Autodesk Fusion 360 part; units mm, degrees
(part 3 of 6)
sketch "b bottom  projection" plane through (0, 0, 0) normal (0, 0, 1) x (1, 0, 0) in component "b bottom component"
  arc A0 (298.8505, 15.08) -> (300.4408, 15.08) centre (299.6456, 15.6946) ccw
  arc A1 (300.4408, 24.92) -> (298.8505, 24.92) centre (299.6456, 24.3054) ccw
  arc A2 (298.835, 24.8994) -> (298.835, 23.7113) centre (299.6456, 24.3054) ccw
  arc A3 (291.9094, 3.175) -> (290.7213, 3.175) centre (291.3154, 2.3644) ccw
  arc A4 (291.93, 1.5692) -> (291.93, 3.1595) centre (291.3154, 2.3644) ccw
  arc A5 (298.835, 36.2887) -> (298.835, 35.1006) centre (299.6456, 35.6946) ccw
  arc A6 (298.8505, 35.08) -> (300.4408, 35.08) centre (299.6456, 35.6946) ccw
  arc A7 (282.09, 3.1595) -> (282.09, 1.5692) centre (282.7046, 2.3644) ccw
  arc A8 (283.2987, 3.175) -> (282.1106, 3.175) centre (282.7046, 2.3644) ccw
  arc A9 (300.4408, 44.92) -> (298.8505, 44.92) centre (299.6456, 44.3054) ccw
  arc A10 (298.835, 44.8994) -> (298.835, 43.7113) centre (299.6456, 44.3054) ccw
  arc A11 (271.9094, 3.175) -> (270.7213, 3.175) centre (271.3154, 2.3644) ccw
  arc A12 (271.93, 1.5692) -> (271.93, 3.1595) centre (271.3154, 2.3644) ccw
  arc A13 (298.835, 56.2887) -> (298.835, 55.1006) centre (299.6456, 55.6946) ccw
  arc A14 (298.8505, 55.08) -> (300.4408, 55.08) centre (299.6456, 55.6946) ccw
  arc A15 (262.09, 3.1595) -> (262.09, 1.5692) centre (262.7046, 2.3644) ccw
  arc A16 (263.2987, 3.175) -> (262.1106, 3.175) centre (262.7046, 2.3644) ccw
  arc A17 (300.4408, 64.92) -> (298.8505, 64.92) centre (299.6456, 64.3054) ccw
  arc A18 (298.835, 64.8994) -> (298.835, 63.7113) centre (299.6456, 64.3054) ccw
  arc A19 (251.9094, 3.175) -> (250.7213, 3.175) centre (251.3154, 2.3644) ccw
  arc A20 (251.93, 1.5692) -> (251.93, 3.1595) centre (251.3154, 2.3644) ccw
  arc A21 (298.835, 76.2887) -> (298.835, 75.1006) centre (299.6456, 75.6946) ccw
  arc A22 (298.8505, 75.08) -> (300.4408, 75.08) centre (299.6456, 75.6946) ccw
  arc A23 (242.09, 3.1595) -> (242.09, 1.5692) centre (242.7046, 2.3644) ccw
  arc A24 (243.2987, 3.175) -> (242.1106, 3.175) centre (242.7046, 2.3644) ccw
  arc A25 (300.4408, 84.92) -> (298.8505, 84.92) centre (299.6456, 84.3054) ccw
  arc A26 (298.835, 84.8994) -> (298.835, 83.7113) centre (299.6456, 84.3054) ccw
  arc A27 (231.9094, 3.175) -> (230.7213, 3.175) centre (231.3154, 2.3644) ccw
  arc A28 (231.93, 1.5692) -> (231.93, 3.1595) centre (231.3154, 2.3644) ccw
  arc A29 (222.09, 3.1595) -> (222.09, 1.5692) centre (222.7046, 2.3644) ccw
  arc A30 (223.2987, 3.175) -> (222.1106, 3.175) centre (222.7046, 2.3644) ccw
  arc A31 (298.835, 96.2887) -> (298.835, 95.1006) centre (299.6456, 95.6946) ccw
  arc A32 (298.8505, 95.08) -> (300.4408, 95.08) centre (299.6456, 95.6946) ccw
  arc A33 (300.4408, 104.92) -> (298.8505, 104.92) centre (299.6456, 104.3054) ccw
  arc A34 (298.835, 104.8994) -> (298.835, 103.7113) centre (299.6456, 104.3054) ccw
  arc A35 (211.9094, 3.175) -> (210.7213, 3.175) centre (211.3154, 2.3644) ccw
  arc A36 (211.93, 1.5692) -> (211.93, 3.1595) centre (211.3154, 2.3644) ccw
  arc A37 (202.09, 3.1595) -> (202.09, 1.5692) centre (202.7046, 2.3644) ccw
  arc A38 (203.2987, 3.175) -> (202.1106, 3.175) centre (202.7046, 2.3644) ccw
  arc A39 (290.7213, 116.825) -> (291.9094, 116.825) centre (291.3154, 117.6356) ccw
  arc A40 (291.93, 116.8405) -> (291.93, 118.4308) centre (291.3154, 117.6356) ccw
  arc A41 (191.9094, 3.175) -> (190.7213, 3.175) centre (191.3154, 2.3644) ccw
  arc A42 (191.93, 1.5692) -> (191.93, 3.1595) centre (191.3154, 2.3644) ccw
  arc A43 (282.09, 118.4308) -> (282.09, 116.8405) centre (282.7046, 117.6356) ccw
  arc A44 (282.1106, 116.825) -> (283.2987, 116.825) centre (282.7046, 117.6356) ccw
  arc A45 (182.09, 3.1595) -> (182.09, 1.5692) centre (182.7046, 2.3644) ccw
  arc A46 (183.2987, 3.175) -> (182.1106, 3.175) centre (182.7046, 2.3644) ccw
  arc A47 (270.7213, 116.825) -> (271.9094, 116.825) centre (271.3154, 117.6356) ccw
  arc A48 (271.93, 116.8405) -> (271.93, 118.4308) centre (271.3154, 117.6356) ccw
  arc A49 (171.9094, 3.175) -> (170.7213, 3.175) centre (171.3154, 2.3644) ccw
  arc A50 (171.93, 1.5692) -> (171.93, 3.1595) centre (171.3154, 2.3644) ccw
  arc A51 (262.09, 118.4308) -> (262.09, 116.8405) centre (262.7046, 117.6356) ccw
  arc A52 (262.1106, 116.825) -> (263.2987, 116.825) centre (262.7046, 117.6356) ccw
  arc A53 (162.09, 3.1595) -> (162.09, 1.5692) centre (162.7046, 2.3644) ccw
  arc A54 (163.2987, 3.175) -> (162.1106, 3.175) centre (162.7046, 2.3644) ccw
  arc A55 (250.7213, 116.825) -> (251.9094, 116.825) centre (251.3154, 117.6356) ccw
  arc A56 (251.93, 116.8405) -> (251.93, 118.4308) centre (251.3154, 117.6356) ccw
  arc A57 (242.09, 118.4308) -> (242.09, 116.8405) centre (242.7046, 117.6356) ccw
  arc A58 (242.1106, 116.825) -> (243.2987, 116.825) centre (242.7046, 117.6356) ccw
  arc A59 (155.185, 15.1006) -> (155.185, 16.2887) centre (154.3744, 15.6946) ccw
  arc A60 (153.5792, 15.08) -> (155.1695, 15.08) centre (154.3744, 15.6946) ccw
  arc A61 (155.1695, 24.92) -> (153.5792, 24.92) centre (154.3744, 24.3054) ccw
  arc A62 (155.185, 23.7113) -> (155.185, 24.8994) centre (154.3744, 24.3054) ccw
  arc A63 (230.7213, 116.825) -> (231.9094, 116.825) centre (231.3154, 117.6356) ccw
  arc A64 (231.93, 116.8405) -> (231.93, 118.4308) centre (231.3154, 117.6356) ccw
  arc A65 (155.185, 35.1006) -> (155.185, 36.2887) centre (154.3744, 35.6946) ccw
  arc A66 (153.5792, 35.08) -> (155.1695, 35.08) centre (154.3744, 35.6946) ccw
  arc A67 (222.09, 118.4308) -> (222.09, 116.8405) centre (222.7046, 117.6356) ccw
  arc A68 (222.1106, 116.825) -> (223.2987, 116.825) centre (222.7046, 117.6356) ccw
  arc A69 (155.1695, 44.92) -> (153.5792, 44.92) centre (154.3744, 44.3054) ccw
  arc A70 (155.185, 43.7113) -> (155.185, 44.8994) centre (154.3744, 44.3054) ccw
  arc A71 (210.7213, 116.825) -> (211.9094, 116.825) centre (211.3154, 117.6356) ccw
  arc A72 (211.93, 116.8405) -> (211.93, 118.4308) centre (211.3154, 117.6356) ccw
  arc A73 (155.185, 55.1006) -> (155.185, 56.2887) centre (154.3744, 55.6946) ccw
  arc A74 (153.5792, 55.08) -> (155.1695, 55.08) centre (154.3744, 55.6946) ccw
  arc A75 (202.09, 118.4308) -> (202.09, 116.8405) centre (202.7046, 117.6356) ccw
  arc A76 (202.1106, 116.825) -> (203.2987, 116.825) centre (202.7046, 117.6356) ccw
  arc A77 (155.1695, 64.92) -> (153.5792, 64.92) centre (154.3744, 64.3054) ccw
  arc A78 (155.185, 63.7113) -> (155.185, 64.8994) centre (154.3744, 64.3054) ccw
  arc A79 (190.7213, 116.825) -> (191.9094, 116.825) centre (191.3154, 117.6356) ccw
  arc A80 (191.93, 116.8405) -> (191.93, 118.4308) centre (191.3154, 117.6356) ccw
  arc A81 (155.185, 75.1006) -> (155.185, 76.2887) centre (154.3744, 75.6946) ccw
  arc A82 (153.5792, 75.08) -> (155.1695, 75.08) centre (154.3744, 75.6946) ccw
  arc A83 (182.09, 118.4308) -> (182.09, 116.8405) centre (182.7046, 117.6356) ccw
  arc A84 (182.1106, 116.825) -> (183.2987, 116.825) centre (182.7046, 117.6356) ccw
  arc A85 (155.1695, 84.92) -> (153.5792, 84.92) centre (154.3744, 84.3054) ccw
  arc A86 (155.185, 83.7113) -> (155.185, 84.8994) centre (154.3744, 84.3054) ccw
  arc A87 (170.7213, 116.825) -> (171.9094, 116.825) centre (171.3154, 117.6356) ccw
  arc A88 (171.93, 116.8405) -> (171.93, 118.4308) centre (171.3154, 117.6356) ccw
  arc A89 (155.185, 95.1006) -> (155.185, 96.2887) centre (154.3744, 95.6946) ccw
  arc A90 (153.5792, 95.08) -> (155.1695, 95.08) centre (154.3744, 95.6946) ccw
  arc A91 (162.09, 118.4308) -> (162.09, 116.8405) centre (162.7046, 117.6356) ccw
  arc A92 (162.1106, 116.825) -> (163.2987, 116.825) centre (162.7046, 117.6356) ccw
  arc A93 (155.1695, 104.92) -> (153.5792, 104.92) centre (154.3744, 104.3054) ccw
  arc A94 (155.185, 103.7113) -> (155.185, 104.8994) centre (154.3744, 104.3054) ccw
  arc A95 (298.835, 16.2887) -> (298.835, 15.1006) centre (299.6456, 15.6946) ccw
  line L0 (302.01, 15.08) -> (300.4408, 15.08)
  line L1 (298.835, 24.8994) -> (298.835, 24.92)
  line L2 (298.835, 16.2887) -> (298.835, 23.7113)
  line L3 (298.835, 15.08) -> (298.835, 15.1006)
  line L4 (300.4408, 24.92) -> (302.01, 24.92)
  line L5 (291.93, 3.175) -> (291.93, 3.1595)
  line L6 (298.8505, 35.08) -> (298.835, 35.08)
  line L7 (282.09, 3.175) -> (282.1106, 3.175)
  line L8 (283.2987, 3.175) -> (290.7213, 3.175)
  line L9 (282.09, 0) -> (282.09, 1.5692)
  line L10 (298.835, 44.8994) -> (298.835, 44.92)
  line L11 (298.835, 36.2887) -> (298.835, 43.7113)
  line L12 (300.4408, 44.92) -> (302.01, 44.92)
  line L13 (271.93, 3.175) -> (271.93, 3.1595)
  line L14 (298.8505, 55.08) -> (298.835, 55.08)
  line L15 (262.09, 3.175) -> (262.1106, 3.175)
  line L16 (263.2987, 3.175) -> (270.7213, 3.175)
  line L17 (262.09, 0) -> (262.09, 1.5692)
  line L18 (298.835, 64.8994) -> (298.835, 64.92)
  line L19 (298.835, 56.2887) -> (298.835, 63.7113)
  line L20 (251.93, 3.175) -> (251.93, 3.1595)
  line L21 (300.4408, 64.92) -> (302.01, 64.92)
  line L22 (298.8505, 75.08) -> (298.835, 75.08)
  line L23 (242.09, 3.175) -> (242.1106, 3.175)
  line L24 (243.2987, 3.175) -> (250.7213, 3.175)
  line L25 (242.09, 0) -> (242.09, 1.5692)
  line L26 (298.835, 84.8994) -> (298.835, 84.92)
  line L27 (298.835, 76.2887) -> (298.835, 83.7113)
  line L28 (231.93, 3.175) -> (231.93, 3.1595)
  line L29 (300.4408, 84.92) -> (302.01, 84.92)
  line L30 (222.09, 3.175) -> (222.1106, 3.175)
  line L31 (223.2987, 3.175) -> (230.7213, 3.175)
  line L32 (298.8505, 95.08) -> (298.835, 95.08)
  line L33 (222.09, 0) -> (222.09, 1.5692)
  line L34 (298.835, 104.8994) -> (298.835, 104.92)
  line L35 (298.835, 96.2887) -> (298.835, 103.7113)
  line L36 (211.93, 3.175) -> (211.93, 3.1595)
  line L37 (300.4408, 104.92) -> (302.01, 104.92)
  line L38 (202.09, 3.175) -> (202.1106, 3.175)
  line L39 (203.2987, 3.175) -> (210.7213, 3.175)
  line L40 (291.93, 116.825) -> (291.93, 116.8405)
  line L41 (202.09, 0) -> (202.09, 1.5692)
  line L42 (282.09, 116.825) -> (282.1106, 116.825)
  line L43 (283.2987, 116.825) -> (290.7213, 116.825)
  line L44 (191.93, 3.175) -> (191.93, 3.1595)
  line L45 (282.09, 120) -> (282.09, 118.4308)
  line L46 (182.09, 3.175) -> (182.1106, 3.175)
  line L47 (183.2987, 3.175) -> (190.7213, 3.175)
  line L48 (271.93, 116.825) -> (271.93, 116.8405)
  line L49 (182.09, 0) -> (182.09, 1.5692)
  line L50 (262.09, 116.825) -> (262.1106, 116.825)
  line L51 (263.2987, 116.825) -> (270.7213, 116.825)
  line L52 (171.93, 3.175) -> (171.93, 3.1595)
  line L53 (262.09, 120) -> (262.09, 118.4308)
  line L54 (162.09, 3.175) -> (162.1106, 3.175)
  line L55 (163.2987, 3.175) -> (170.7213, 3.175)
  line L56 (251.93, 116.825) -> (251.93, 116.8405)
  line L57 (162.09, 0) -> (162.09, 1.5692)
  line L58 (242.09, 116.825) -> (242.1106, 116.825)
  line L59 (243.2987, 116.825) -> (250.7213, 116.825)
  line L60 (155.1695, 15.08) -> (155.185, 15.08)
  line L61 (242.09, 120) -> (242.09, 118.4308)
  line L62 (155.185, 24.8994) -> (155.185, 24.92)
  line L63 (155.185, 16.2887) -> (155.185, 23.7113)
  line L64 (231.93, 116.825) -> (231.93, 116.8405)
  line L65 (153.5792, 24.92) -> (152.01, 24.92)
  line L66 (222.09, 116.825) -> (222.1106, 116.825)
  line L67 (223.2987, 116.825) -> (230.7213, 116.825)
  line L68 (155.1695, 35.08) -> (155.185, 35.08)
  line L69 (222.09, 120) -> (222.09, 118.4308)
  line L70 (155.185, 44.8994) -> (155.185, 44.92)
  line L71 (155.185, 36.2887) -> (155.185, 43.7113)
  line L72 (211.93, 116.825) -> (211.93, 116.8405)
  line L73 (153.5792, 44.92) -> (152.01, 44.92)
  line L74 (155.1695, 55.08) -> (155.185, 55.08)
  line L75 (202.09, 116.825) -> (202.1106, 116.825)
  line L76 (203.2987, 116.825) -> (210.7213, 116.825)
  line L77 (202.09, 120) -> (202.09, 118.4308)
  line L78 (155.185, 64.8994) -> (155.185, 64.92)
  line L79 (155.185, 56.2887) -> (155.185, 63.7113)
  line L80 (153.5792, 64.92) -> (152.01, 64.92)
  line L81 (191.93, 116.825) -> (191.93, 116.8405)
  line L82 (155.1695, 75.08) -> (155.185, 75.08)
  line L83 (182.09, 116.825) -> (182.1106, 116.825)
  line L84 (183.2987, 116.825) -> (190.7213, 116.825)
  line L85 (155.185, 84.8994) -> (155.185, 84.92)
  line L86 (155.185, 76.2887) -> (155.185, 83.7113)
  line L87 (182.09, 120) -> (182.09, 118.4308)
  line L88 (153.5792, 84.92) -> (152.01, 84.92)
  line L89 (171.93, 116.825) -> (171.93, 116.8405)
  line L90 (155.1695, 95.08) -> (155.185, 95.08)
  line L91 (162.09, 116.825) -> (162.1106, 116.825)
  line L92 (163.2987, 116.825) -> (170.7213, 116.825)
  line L93 (155.185, 104.8994) -> (155.185, 104.92)
  line L94 (155.185, 96.2887) -> (155.185, 103.7113)
  line L95 (162.09, 120) -> (162.09, 118.4308)
  line L96 (153.5792, 104.92) -> (152.01, 104.92)
  line L97 (152.01, 0) -> (152.01, 15.08)
  line L98 (152.01, 15.08) -> (153.5792, 15.08)
  line L99 (155.185, 15.08) -> (155.185, 15.1006)
  line L100 (155.185, 24.92) -> (155.1695, 24.92)
  line L101 (152.01, 24.92) -> (152.01, 35.08)
  line L102 (152.01, 35.08) -> (153.5792, 35.08)
  line L103 (155.185, 35.08) -> (155.185, 35.1006)
  line L104 (155.185, 44.92) -> (155.1695, 44.92)
  line L105 (152.01, 44.92) -> (152.01, 55.08)
  line L106 (152.01, 55.08) -> (153.5792, 55.08)
  line L107 (155.185, 55.08) -> (155.185, 55.1006)
  line L108 (155.185, 64.92) -> (155.1695, 64.92)
  line L109 (152.01, 64.92) -> (152.01, 75.08)
  line L110 (152.01, 75.08) -> (153.5792, 75.08)
  line L111 (155.185, 75.08) -> (155.185, 75.1006)
  line L112 (155.185, 84.92) -> (155.1695, 84.92)
  line L113 (152.01, 84.92) -> (152.01, 95.08)
  line L114 (152.01, 95.08) -> (153.5792, 95.08)
  line L115 (155.185, 95.08) -> (155.185, 95.1006)
  line L116 (155.185, 104.92) -> (155.1695, 104.92)
  line L117 (152.01, 104.92) -> (152.01, 120)
  line L118 (152.01, 120) -> (162.09, 120)
  line L119 (162.09, 116.8405) -> (162.09, 116.825)
  line L120 (171.9094, 116.825) -> (171.93, 116.825)
  line L121 (171.93, 118.4308) -> (171.93, 120)
  line L122 (171.93, 120) -> (182.09, 120)
  line L123 (182.09, 116.8405) -> (182.09, 116.825)
  line L124 (191.9094, 116.825) -> (191.93, 116.825)
  line L125 (191.93, 118.4308) -> (191.93, 120)
  line L126 (191.93, 120) -> (202.09, 120)
  line L127 (202.09, 116.8405) -> (202.09, 116.825)
  line L128 (211.9094, 116.825) -> (211.93, 116.825)
  line L129 (211.93, 118.4308) -> (211.93, 120)
  line L130 (211.93, 120) -> (222.09, 120)
  line L131 (222.09, 116.8405) -> (222.09, 116.825)
  line L132 (231.9094, 116.825) -> (231.93, 116.825)
  line L133 (231.93, 118.4308) -> (231.93, 120)
  line L134 (231.93, 120) -> (242.09, 120)
  line L135 (242.09, 116.8405) -> (242.09, 116.825)
  line L136 (251.9094, 116.825) -> (251.93, 116.825)
  line L137 (251.93, 118.4308) -> (251.93, 120)
  line L138 (251.93, 120) -> (262.09, 120)
  line L139 (262.09, 116.8405) -> (262.09, 116.825)
  line L140 (271.9094, 116.825) -> (271.93, 116.825)
  line L141 (271.93, 118.4308) -> (271.93, 120)
  line L142 (271.93, 120) -> (282.09, 120)
  line L143 (282.09, 116.8405) -> (282.09, 116.825)
  line L144 (291.9094, 116.825) -> (291.93, 116.825)
  line L145 (291.93, 118.4308) -> (291.93, 120)
  line L146 (291.93, 120) -> (302.01, 120)
  line L147 (302.01, 104.92) -> (302.01, 120)
  line L148 (298.835, 104.92) -> (298.8505, 104.92)
  line L149 (298.835, 95.08) -> (298.835, 95.1006)
  line L150 (302.01, 95.08) -> (300.4408, 95.08)
  line L151 (302.01, 84.92) -> (302.01, 95.08)
  line L152 (298.835, 84.92) -> (298.8505, 84.92)
  line L153 (298.835, 75.08) -> (298.835, 75.1006)
  line L154 (302.01, 75.08) -> (300.4408, 75.08)
  line L155 (302.01, 64.92) -> (302.01, 75.08)
  line L156 (298.835, 64.92) -> (298.8505, 64.92)
  line L157 (298.835, 55.08) -> (298.835, 55.1006)
  line L158 (302.01, 55.08) -> (300.4408, 55.08)
  line L159 (302.01, 44.92) -> (302.01, 55.08)
  line L160 (298.835, 44.92) -> (298.8505, 44.92)
  line L161 (298.835, 35.08) -> (298.835, 35.1006)
  line L162 (302.01, 35.08) -> (300.4408, 35.08)
  line L163 (302.01, 24.92) -> (302.01, 35.08)
  line L164 (298.835, 24.92) -> (298.8505, 24.92)
  line L165 (298.8505, 15.08) -> (298.835, 15.08)
  line L166 (302.01, 0) -> (302.01, 15.08)
  line L167 (291.93, 0) -> (302.01, 0)
  line L168 (291.93, 1.5692) -> (291.93, 0)
  line L169 (291.9094, 3.175) -> (291.93, 3.175)
  line L170 (282.09, 3.1595) -> (282.09, 3.175)
  line L171 (271.93, 0) -> (282.09, 0)
  line L172 (271.93, 1.5692) -> (271.93, 0)
  line L173 (271.9094, 3.175) -> (271.93, 3.175)
  line L174 (262.09, 3.1595) -> (262.09, 3.175)
  line L175 (251.93, 0) -> (262.09, 0)
  line L176 (251.93, 1.5692) -> (251.93, 0)
  line L177 (251.9094, 3.175) -> (251.93, 3.175)
  line L178 (242.09, 3.1595) -> (242.09, 3.175)
  line L179 (231.93, 0) -> (242.09, 0)
  line L180 (231.93, 1.5692) -> (231.93, 0)
  line L181 (231.9094, 3.175) -> (231.93, 3.175)
  line L182 (222.09, 3.1595) -> (222.09, 3.175)
  line L183 (211.93, 0) -> (222.09, 0)
  line L184 (211.93, 1.5692) -> (211.93, 0)
  line L185 (211.9094, 3.175) -> (211.93, 3.175)
  line L186 (202.09, 3.1595) -> (202.09, 3.175)
  line L187 (191.93, 0) -> (202.09, 0)
  line L188 (191.93, 1.5692) -> (191.93, 0)
  line L189 (191.9094, 3.175) -> (191.93, 3.175)
  line L190 (182.09, 3.1595) -> (182.09, 3.175)
  line L191 (171.93, 0) -> (182.09, 0)
  line L192 (171.93, 1.5692) -> (171.93, 0)
  line L193 (171.9094, 3.175) -> (171.93, 3.175)
  line L194 (162.09, 3.1595) -> (162.09, 3.175)
  line L195 (152.01, 0) -> (162.09, 0)
sketch "b front lines" plane through (0, 0, 0) normal (0, 0, 1) x (1, 0, 0) in component "b front component"
  line L0 (3.175, 125.185) -> (9.92, 125.185)
  line L1 (9.92, 125.185) -> (9.92, 122.01)
  line L2 (9.92, 122.01) -> (20.08, 122.01)
  line L3 (20.08, 122.01) -> (20.08, 125.185)
  line L4 (20.08, 125.185) -> (29.92, 125.185)
  line L5 (29.92, 125.185) -> (29.92, 122.01)
  line L6 (29.92, 122.01) -> (40.08, 122.01)
  line L7 (40.08, 122.01) -> (40.08, 125.185)
  line L8 (40.08, 125.185) -> (49.92, 125.185)
  line L9 (49.92, 125.185) -> (49.92, 122.01)
  line L10 (49.92, 122.01) -> (60.08, 122.01)
  line L11 (60.08, 122.01) -> (60.08, 125.185)
  line L12 (60.08, 125.185) -> (69.92, 125.185)
  line L13 (69.92, 125.185) -> (69.92, 122.01)
  line L14 (69.92, 122.01) -> (80.08, 122.01)
  line L15 (80.08, 122.01) -> (80.08, 125.185)
  line L16 (80.08, 125.185) -> (89.92, 125.185)
  line L17 (89.92, 125.185) -> (89.92, 122.01)
  line L18 (89.92, 122.01) -> (100.08, 122.01)
  line L19 (100.08, 122.01) -> (100.08, 125.185)
  line L20 (100.08, 125.185) -> (109.92, 125.185)
  line L21 (109.92, 125.185) -> (109.92, 122.01)
  line L22 (109.92, 122.01) -> (120.08, 122.01)
  line L23 (120.08, 122.01) -> (120.08, 125.185)
  line L24 (120.08, 125.185) -> (129.92, 125.185)
  line L25 (129.92, 125.185) -> (129.92, 122.01)
  line L26 (129.92, 122.01) -> (140.08, 122.01)
  line L27 (140.08, 122.01) -> (140.08, 125.185)
  line L28 (140.08, 125.185) -> (146.825, 125.185)
  line L29 (146.825, 125.185) -> (146.825, 139.43)
  line L30 (146.825, 139.43) -> (150, 139.43)
  line L31 (150, 139.43) -> (150, 149.59)
  line L32 (150, 149.59) -> (146.825, 149.59)
  line L33 (146.825, 149.59) -> (146.825, 159.43)
  line L34 (146.825, 159.43) -> (150, 159.43)
  line L35 (150, 159.43) -> (150, 169.59)
  line L36 (150, 169.59) -> (146.825, 169.59)
  line L37 (146.825, 169.59) -> (146.825, 183.835)
  line L38 (3.175, 183.835) -> (9.92, 183.835)
  line L39 (9.92, 183.835) -> (9.92, 187.01)
  line L40 (9.92, 187.01) -> (20.08, 187.01)
  line L41 (20.08, 187.01) -> (20.08, 183.835)
  line L42 (20.08, 183.835) -> (29.92, 183.835)
  line L43 (29.92, 183.835) -> (29.92, 187.01)
  line L44 (29.92, 187.01) -> (40.08, 187.01)
  line L45 (40.08, 187.01) -> (40.08, 183.835)
  line L46 (40.08, 183.835) -> (49.92, 183.835)
  line L47 (49.92, 183.835) -> (49.92, 187.01)
  line L48 (49.92, 187.01) -> (60.08, 187.01)
  line L49 (60.08, 187.01) -> (60.08, 183.835)
  line L50 (60.08, 183.835) -> (69.92, 183.835)
  line L51 (69.92, 183.835) -> (69.92, 187.01)
  line L52 (69.92, 187.01) -> (80.08, 187.01)
  line L53 (80.08, 187.01) -> (80.08, 183.835)
  line L54 (80.08, 183.835) -> (89.92, 183.835)
  line L55 (89.92, 183.835) -> (89.92, 187.01)
  line L56 (89.92, 187.01) -> (100.08, 187.01)
  line L57 (100.08, 187.01) -> (100.08, 183.835)
  line L58 (100.08, 183.835) -> (109.92, 183.835)
  line L59 (109.92, 183.835) -> (109.92, 187.01)
  line L60 (109.92, 187.01) -> (120.08, 187.01)
  line L61 (120.08, 187.01) -> (120.08, 183.835)
  line L62 (120.08, 183.835) -> (129.92, 183.835)
  line L63 (129.92, 183.835) -> (129.92, 187.01)
  line L64 (129.92, 187.01) -> (140.08, 187.01)
  line L65 (140.08, 187.01) -> (140.08, 183.835)
  line L66 (140.08, 183.835) -> (146.825, 183.835)
  line L67 (3.175, 125.185) -> (3.175, 139.43)
  line L68 (3.175, 139.43) -> (0, 139.43)
  line L69 (0, 139.43) -> (0, 149.59)
  line L70 (0, 149.59) -> (3.175, 149.59)
  line L71 (3.175, 149.59) -> (3.175, 159.43)
  line L72 (3.175, 159.43) -> (0, 159.43)
  line L73 (0, 159.43) -> (0, 169.59)
  line L74 (0, 169.59) -> (3.175, 169.59)
  line L75 (3.175, 169.59) -> (3.175, 183.835)
  dimension "d5494" = 6.745
  dimension "d5495" = 3.175
  dimension "d5496" = 10.16
  dimension "d5497" = 3.175
  dimension "d5498" = 9.84
  dimension "d5499" = 3.175
  dimension "d5500" = 10.16
  dimension "d5501" = 3.175
  dimension "d5502" = 9.84
  dimension "d5503" = 3.175
  dimension "d5504" = 10.16
  dimension "d5505" = 3.175
  dimension "d5506" = 9.84
  dimension "d5507" = 3.175
  dimension "d5508" = 10.16
  dimension "d5509" = 3.175
  dimension "d5510" = 9.84
  dimension "d5511" = 3.175
  dimension "d5512" = 10.16
  dimension "d5513" = 3.175
  dimension "d5514" = 9.84
  dimension "d5515" = 3.175
  dimension "d5516" = 10.16
  dimension "d5517" = 3.175
  dimension "d5518" = 9.84
  dimension "d5519" = 3.175
  dimension "d5520" = 10.16
  dimension "d5521" = 3.175
  dimension "d5522" = 6.745
  dimension "d5537" = 14.245
  dimension "d5538" = 3.175
  dimension "d5539" = 10.16
  dimension "d5540" = 3.175
  dimension "d5541" = 9.84
  dimension "d5542" = 3.175
  dimension "d5543" = 10.16
  dimension "d5544" = 3.175
  dimension "d5545" = 14.245
  dimension "d5550" = 6.745
  dimension "d5551" = 3.175
  dimension "d5552" = 10.16
  dimension "d5553" = 3.175
  dimension "d5554" = 9.84
  dimension "d5555" = 3.175
  dimension "d5556" = 10.16
  dimension "d5557" = 3.175
  dimension "d5558" = 9.84
  dimension "d5559" = 3.175
  dimension "d5560" = 10.16
  dimension "d5561" = 3.175
  dimension "d5562" = 9.84
  dimension "d5563" = 3.175
  dimension "d5564" = 10.16
  dimension "d5565" = 3.175
  dimension "d5566" = 9.84
  dimension "d5567" = 3.175
  dimension "d5568" = 10.16
  dimension "d5569" = 3.175
  dimension "d5570" = 9.84
  dimension "d5571" = 3.175
  dimension "d5572" = 10.16
  dimension "d5573" = 3.175
  dimension "d5574" = 9.84
  dimension "d5575" = 3.175
  dimension "d5576" = 10.16
  dimension "d5577" = 3.175
  dimension "d5578" = 6.745
  dimension "d5593" = 14.245
  dimension "d5594" = 3.175
  dimension "d5595" = 10.16
  dimension "d5596" = 3.175
  dimension "d5597" = 9.84
  dimension "d5598" = 3.175
  dimension "d5599" = 10.16
  dimension "d5600" = 3.175
  dimension "d5601" = 14.245
  constraint horizontal L0
  constraint vertical L1
  constraint horizontal L2
  constraint vertical L3
  constraint horizontal L4
  constraint vertical L5
  constraint horizontal L6
  constraint vertical L7
  constraint horizontal L8
  constraint vertical L9
  constraint horizontal L10
  constraint vertical L11
  constraint horizontal L12
  constraint vertical L13
  constraint horizontal L14
  constraint vertical L15
  constraint horizontal L16
  constraint vertical L17
  constraint horizontal L18
  constraint vertical L19
  constraint horizontal L20
  constraint vertical L21
  constraint horizontal L22
  constraint vertical L23
  constraint horizontal L24
  constraint vertical L25
  constraint horizontal L26
  constraint vertical L27
  constraint horizontal L28
  constraint vertical L29
  constraint horizontal L30
  constraint vertical L31
  constraint horizontal L32
  constraint vertical L33
  constraint horizontal L34
  constraint vertical L35
  constraint horizontal L36
  constraint vertical L37
  constraint horizontal L38
  constraint vertical L39
  constraint horizontal L40
  constraint vertical L41
  constraint horizontal L42
  constraint vertical L43
  constraint horizontal L44
  constraint vertical L45
  constraint horizontal L46
  constraint vertical L47
  constraint horizontal L48
  constraint vertical L49
  constraint horizontal L50
  constraint vertical L51
  constraint horizontal L52
  constraint vertical L53
  constraint horizontal L54
  constraint vertical L55
  constraint horizontal L56
  constraint vertical L57
  constraint horizontal L58
  constraint vertical L59
  constraint horizontal L60
  constraint vertical L61
  constraint horizontal L62
  constraint vertical L63
  constraint horizontal L64
  constraint vertical L65
  constraint horizontal L66
  constraint vertical L67
  constraint horizontal L68
  constraint vertical L69
  constraint horizontal L70
  constraint vertical L71
  constraint horizontal L72
  constraint vertical L73
  constraint horizontal L74
  constraint vertical L75
  measures "d5494" distance of L0.start L0.end
  measures "d5495" distance of L0.end L1.end
  measures "d5496" distance of L1.end L2.end
  measures "d5497" distance of L2.end L3.end
  measures "d5498" distance of L3.end L4.end
  measures "d5499" distance of L4.end L5.end
  measures "d5500" distance of L5.end L6.end
  measures "d5501" distance of L6.end L7.end
  measures "d5502" distance of L7.end L8.end
  measures "d5503" distance of L8.end L9.end
  measures "d5504" distance of L9.end L10.end
  measures "d5505" distance of L10.end L11.end
  measures "d5506" distance of L11.end L12.end
  measures "d5507" distance of L12.end L13.end
  measures "d5508" distance of L13.end L14.end
  measures "d5509" distance of L14.end L15.end
  measures "d5510" distance of L15.end L16.end
  measures "d5511" distance of L16.end L17.end
  measures "d5512" distance of L17.end L18.end
  measures "d5513" distance of L18.end L19.end
  measures "d5514" distance of L19.end L20.end
  measures "d5515" distance of L20.end L21.end
  measures "d5516" distance of L21.end L22.end
  measures "d5517" distance of L22.end L23.end
  measures "d5518" distance of L23.end L24.end
  measures "d5519" distance of L24.end L25.end
  measures "d5520" distance of L25.end L26.end
  measures "d5521" distance of L26.end L27.end
  measures "d5522" distance of L27.end L28.end
  measures "d5537" distance of L28.end L29.end
  measures "d5538" distance of L29.end L30.end
  measures "d5539" distance of L30.end L31.end
  measures "d5540" distance of L31.end L32.end
  measures "d5541" distance of L32.end L33.end
  measures "d5542" distance of L33.end L34.end
  measures "d5543" distance of L34.end L35.end
  measures "d5544" distance of L35.end L36.end
  measures "d5545" distance of L36.end L37.end
  measures "d5550" distance of L38.start L38.end
  measures "d5551" distance of L38.end L39.end
  measures "d5552" distance of L39.end L40.end
  measures "d5553" distance of L40.end L41.end
  measures "d5554" distance of L41.end L42.end
  measures "d5555" distance of L42.end L43.end
  measures "d5556" distance of L43.end L44.end
  measures "d5557" distance of L44.end L45.end
  measures "d5558" distance of L45.end L46.end
  measures "d5559" distance of L46.end L47.end
  measures "d5560" distance of L47.end L48.end
  measures "d5561" distance of L48.end L49.end
  measures "d5562" distance of L49.end L50.end
  measures "d5563" distance of L50.end L51.end
  measures "d5564" distance of L51.end L52.end
  measures "d5565" distance of L52.end L53.end
  measures "d5566" distance of L53.end L54.end
  measures "d5567" distance of L54.end L55.end
  measures "d5568" distance of L55.end L56.end
  measures "d5569" distance of L56.end L57.end
  measures "d5570" distance of L57.end L58.end
  measures "d5571" distance of L58.end L59.end
  measures "d5572" distance of L59.end L60.end
  measures "d5573" distance of L60.end L61.end
  measures "d5574" distance of L61.end L62.end
  measures "d5575" distance of L62.end L63.end
  measures "d5576" distance of L63.end L64.end
  measures "d5577" distance of L64.end L65.end
  measures "d5578" distance of L37.end L65.end
  measures "d5593" distance of L0.start L67.end
  measures "d5594" distance of L67.end L68.end
  measures "d5595" distance of L68.end L69.end
  measures "d5596" distance of L69.end L70.end
  measures "d5597" distance of L70.end L71.end
  measures "d5598" distance of L71.end L72.end
  measures "d5599" distance of L72.end L73.end
  measures "d5600" distance of L73.end L74.end
  measures "d5601" distance of L38.start L74.end
sketch "b front circles" plane through (0, 0, 0) normal (0, 0, 1) x (1, 0, 0) in component "b front component"
  line L0 (0, 122.01) -> (150, 122.01)
  line L1 (150, 122.01) -> (150, 187.01)
  line L2 (150, 187.01) -> (0, 187.01)
  line L3 (0, 187.01) -> (0, 122.01)
  circle A0 centre (9.3054, 124.3744) radius 1.005
  circle A1 centre (20.6946, 124.3744) radius 1.005
  circle A2 centre (29.3054, 124.3744) radius 1.005
  circle A3 centre (40.6946, 124.3744) radius 1.005
  circle A4 centre (49.3054, 124.3744) radius 1.005
  circle A5 centre (60.6946, 124.3744) radius 1.005
  circle A6 centre (69.3054, 124.3744) radius 1.005
  circle A7 centre (80.6946, 124.3744) radius 1.005
  circle A8 centre (89.3054, 124.3744) radius 1.005
  circle A9 centre (100.6946, 124.3744) radius 1.005
  circle A10 centre (109.3054, 124.3744) radius 1.005
  circle A11 centre (120.6946, 124.3744) radius 1.005
  circle A12 centre (129.3054, 124.3744) radius 1.005
  circle A13 centre (140.6946, 124.3744) radius 1.005
  circle A14 centre (147.6356, 138.8154) radius 1.005
  circle A15 centre (147.6356, 150.2046) radius 1.005
  circle A16 centre (147.6356, 158.8154) radius 1.005
  circle A17 centre (147.6356, 170.2046) radius 1.005
  circle A18 centre (9.3054, 184.6456) radius 1.005
  circle A19 centre (20.6946, 184.6456) radius 1.005
  circle A20 centre (29.3054, 184.6456) radius 1.005
  circle A21 centre (40.6946, 184.6456) radius 1.005
  circle A22 centre (49.3054, 184.6456) radius 1.005
  circle A23 centre (60.6946, 184.6456) radius 1.005
  circle A24 centre (69.3054, 184.6456) radius 1.005
  circle A25 centre (80.6946, 184.6456) radius 1.005
  circle A26 centre (89.3054, 184.6456) radius 1.005
  circle A27 centre (100.6946, 184.6456) radius 1.005
  circle A28 centre (109.3054, 184.6456) radius 1.005
  circle A29 centre (120.6946, 184.6456) radius 1.005
  circle A30 centre (129.3054, 184.6456) radius 1.005
  circle A31 centre (140.6946, 184.6456) radius 1.005
  circle A32 centre (2.3644, 138.8154) radius 1.005
  circle A33 centre (2.3644, 150.2046) radius 1.005
  circle A34 centre (2.3644, 158.8154) radius 1.005
  circle A35 centre (2.3644, 170.2046) radius 1.005
  dimension "d5523" = 2.01
  dimension "d5524" = 2.01
  dimension "d5525" = 2.01
  dimension "d5526" = 2.01
  dimension "d5527" = 2.01
  dimension "d5528" = 2.01
  dimension "d5529" = 2.01
  dimension "d5530" = 2.01
  dimension "d5531" = 2.01
  dimension "d5532" = 2.01
  dimension "d5533" = 2.01
  dimension "d5534" = 2.01
  dimension "d5535" = 2.01
  dimension "d5536" = 2.01
  dimension "d5546" = 2.01
  dimension "d5547" = 2.01
  dimension "d5548" = 2.01
  dimension "d5549" = 2.01
  dimension "d5579" = 2.01
  dimension "d5580" = 2.01
  dimension "d5581" = 2.01
  dimension "d5582" = 2.01
  dimension "d5583" = 2.01
  dimension "d5584" = 2.01
  dimension "d5585" = 2.01
  dimension "d5586" = 2.01
  dimension "d5587" = 2.01
  dimension "d5588" = 2.01
  dimension "d5589" = 2.01
  dimension "d5590" = 2.01
  dimension "d5591" = 2.01
  dimension "d5592" = 2.01
  dimension "d5602" = 2.01
  dimension "d5603" = 2.01
  dimension "d5604" = 2.01
  dimension "d5605" = 2.01
  measures "d5523" diameter of A0
  measures "d5524" diameter of A1
  measures "d5525" diameter of A2
  measures "d5526" diameter of A3
  measures "d5527" diameter of A4
  measures "d5528" diameter of A5
  measures "d5529" diameter of A6
  measures "d5530" diameter of A7
  measures "d5531" diameter of A8
  measures "d5532" diameter of A9
  measures "d5533" diameter of A10
  measures "d5534" diameter of A11
  measures "d5535" diameter of A12
  measures "d5536" diameter of A13
  measures "d5546" diameter of A14
  measures "d5547" diameter of A15
  measures "d5548" diameter of A16
  measures "d5549" diameter of A17
  measures "d5579" diameter of A18
  measures "d5580" diameter of A19
  measures "d5581" diameter of A20
  measures "d5582" diameter of A21
  measures "d5583" diameter of A22
  measures "d5584" diameter of A23
  measures "d5585" diameter of A24
  measures "d5586" diameter of A25
  measures "d5587" diameter of A26
  measures "d5588" diameter of A27
  measures "d5589" diameter of A28
  measures "d5590" diameter of A29
  measures "d5591" diameter of A30
  measures "d5592" diameter of A31
  measures "d5602" diameter of A32
  measures "d5603" diameter of A33
  measures "d5604" diameter of A34
  measures "d5605" diameter of A35
extrude "b front lines body extrude" add sketch "b front lines" along normal blind 3.175 separate body makes body 6 in component "b front component"
extrude "b front circles extrude" add sketch "b front circles" along normal blind 3.175 separate body makes body 7 in component "b front component"
combine "b front lines final combine feature" operation intersect target body 6 tool bodies 7 in component "b front component"
sketch "b front  projection" plane through (0, 0, 0) normal (0, 0, 1) x (1, 0, 0) in component "b front component"
  arc A0 (146.825, 150.7987) -> (146.825, 149.6106) centre (147.6356, 150.2046) ccw
  arc A1 (146.825, 139.4094) -> (146.825, 138.2213) centre (147.6356, 138.8154) ccw
  arc A2 (148.4308, 159.43) -> (146.8405, 159.43) centre (147.6356, 158.8154) ccw
  arc A3 (140.08, 125.1695) -> (140.08, 123.5792) centre (140.6946, 124.3744) ccw
  arc A4 (146.825, 170.7987) -> (146.825, 169.6106) centre (147.6356, 170.2046) ccw
  arc A5 (129.8994, 125.185) -> (128.7113, 125.185) centre (129.3054, 124.3744) ccw
  arc A6 (140.08, 185.4408) -> (140.08, 183.8505) centre (140.6946, 184.6456) ccw
  arc A7 (120.08, 125.1695) -> (120.08, 123.5792) centre (120.6946, 124.3744) ccw
  arc A8 (128.7113, 183.835) -> (129.8994, 183.835) centre (129.3054, 184.6456) ccw
  arc A9 (109.8994, 125.185) -> (108.7113, 125.185) centre (109.3054, 124.3744) ccw
  arc A10 (120.08, 185.4408) -> (120.08, 183.8505) centre (120.6946, 184.6456) ccw
  arc A11 (100.08, 125.1695) -> (100.08, 123.5792) centre (100.6946, 124.3744) ccw
  arc A12 (108.7113, 183.835) -> (109.8994, 183.835) centre (109.3054, 184.6456) ccw
  arc A13 (89.8994, 125.185) -> (88.7113, 125.185) centre (89.3054, 124.3744) ccw
  arc A14 (100.08, 185.4408) -> (100.08, 183.8505) centre (100.6946, 184.6456) ccw
  arc A15 (80.08, 125.1695) -> (80.08, 123.5792) centre (80.6946, 124.3744) ccw
  arc A16 (88.7113, 183.835) -> (89.8994, 183.835) centre (89.3054, 184.6456) ccw
  arc A17 (69.8994, 125.185) -> (68.7113, 125.185) centre (69.3054, 124.3744) ccw
  arc A18 (80.08, 185.4408) -> (80.08, 183.8505) centre (80.6946, 184.6456) ccw
  arc A19 (60.08, 125.1695) -> (60.08, 123.5792) centre (60.6946, 124.3744) ccw
  arc A20 (68.7113, 183.835) -> (69.8994, 183.835) centre (69.3054, 184.6456) ccw
  arc A21 (49.8994, 125.185) -> (48.7113, 125.185) centre (49.3054, 124.3744) ccw
  arc A22 (60.08, 185.4408) -> (60.08, 183.8505) centre (60.6946, 184.6456) ccw
  arc A23 (40.08, 125.1695) -> (40.08, 123.5792) centre (40.6946, 124.3744) ccw
  arc A24 (48.7113, 183.835) -> (49.8994, 183.835) centre (49.3054, 184.6456) ccw
  arc A25 (29.8994, 125.185) -> (28.7113, 125.185) centre (29.3054, 124.3744) ccw
  arc A26 (40.08, 185.4408) -> (40.08, 183.8505) centre (40.6946, 184.6456) ccw
  arc A27 (20.08, 125.1695) -> (20.08, 123.5792) centre (20.6946, 124.3744) ccw
  arc A28 (28.7113, 183.835) -> (29.8994, 183.835) centre (29.3054, 184.6456) ccw
  arc A29 (9.8994, 125.185) -> (8.7113, 125.185) centre (9.3054, 124.3744) ccw
  arc A30 (20.08, 185.4408) -> (20.08, 183.8505) centre (20.6946, 184.6456) ccw
  arc A31 (3.1595, 139.43) -> (1.5692, 139.43) centre (2.3644, 138.8154) ccw
  arc A32 (8.7113, 183.835) -> (9.8994, 183.835) centre (9.3054, 184.6456) ccw
  arc A33 (3.175, 149.6106) -> (3.175, 150.7987) centre (2.3644, 150.2046) ccw
  arc A34 (3.1595, 159.43) -> (1.5692, 159.43) centre (2.3644, 158.8154) ccw
  arc A35 (1.5692, 169.59) -> (3.1595, 169.59) centre (2.3644, 170.2046) ccw
  arc A36 (120.1006, 183.835) -> (121.2887, 183.835) centre (120.6946, 184.6456) ccw
  arc A37 (129.92, 183.8505) -> (129.92, 185.4408) centre (129.3054, 184.6456) ccw
  arc A38 (140.1006, 183.835) -> (141.2887, 183.835) centre (140.6946, 184.6456) ccw
  arc A39 (3.175, 138.2213) -> (3.175, 139.4094) centre (2.3644, 138.8154) ccw
  arc A40 (1.5692, 149.59) -> (3.1595, 149.59) centre (2.3644, 150.2046) ccw
  arc A41 (3.175, 158.2213) -> (3.175, 159.4094) centre (2.3644, 158.8154) ccw
  arc A42 (3.175, 169.6106) -> (3.175, 170.7987) centre (2.3644, 170.2046) ccw
  arc A43 (101.2887, 125.185) -> (100.1006, 125.185) centre (100.6946, 124.3744) ccw
  arc A44 (21.2887, 125.185) -> (20.1006, 125.185) centre (20.6946, 124.3744) ccw
  arc A45 (29.92, 123.5792) -> (29.92, 125.1695) centre (29.3054, 124.3744) ccw
  arc A46 (49.92, 123.5792) -> (49.92, 125.1695) centre (49.3054, 124.3744) ccw
  arc A47 (129.92, 123.5792) -> (129.92, 125.1695) centre (129.3054, 124.3744) ccw
  arc A48 (60.1006, 183.835) -> (61.2887, 183.835) centre (60.6946, 184.6456) ccw
  arc A49 (89.92, 183.8505) -> (89.92, 185.4408) centre (89.3054, 184.6456) ccw
  arc A50 (100.1006, 183.835) -> (101.2887, 183.835) centre (100.6946, 184.6456) ccw
  arc A51 (80.1006, 183.835) -> (81.2887, 183.835) centre (80.6946, 184.6456) ccw
  arc A52 (69.92, 183.8505) -> (69.92, 185.4408) centre (69.3054, 184.6456) ccw
  arc A53 (146.8405, 149.59) -> (148.4308, 149.59) centre (147.6356, 150.2046) ccw
  arc A54 (81.2887, 125.185) -> (80.1006, 125.185) centre (80.6946, 124.3744) ccw
  arc A55 (41.2887, 125.185) -> (40.1006, 125.185) centre (40.6946, 124.3744) ccw
  arc A56 (121.2887, 125.185) -> (120.1006, 125.185) centre (120.6946, 124.3744) ccw
  arc A57 (146.8405, 169.59) -> (148.4308, 169.59) centre (147.6356, 170.2046) ccw
  arc A58 (20.1006, 183.835) -> (21.2887, 183.835) centre (20.6946, 184.6456) ccw
  arc A59 (9.92, 183.8505) -> (9.92, 185.4408) centre (9.3054, 184.6456) ccw
  arc A60 (141.2887, 125.185) -> (140.1006, 125.185) centre (140.6946, 124.3744) ccw
  arc A61 (61.2887, 125.185) -> (60.1006, 125.185) centre (60.6946, 124.3744) ccw
  arc A62 (9.92, 123.5792) -> (9.92, 125.1695) centre (9.3054, 124.3744) ccw
  arc A63 (89.92, 123.5792) -> (89.92, 125.1695) centre (89.3054, 124.3744) ccw
  arc A64 (146.825, 159.4094) -> (146.825, 158.2213) centre (147.6356, 158.8154) ccw
  arc A65 (40.1006, 183.835) -> (41.2887, 183.835) centre (40.6946, 184.6456) ccw
  arc A66 (29.92, 183.8505) -> (29.92, 185.4408) centre (29.3054, 184.6456) ccw
  arc A67 (69.92, 123.5792) -> (69.92, 125.1695) centre (69.3054, 124.3744) ccw
  arc A68 (109.92, 123.5792) -> (109.92, 125.1695) centre (109.3054, 124.3744) ccw
  arc A69 (148.4308, 139.43) -> (146.8405, 139.43) centre (147.6356, 138.8154) ccw
  arc A70 (49.92, 183.8505) -> (49.92, 185.4408) centre (49.3054, 184.6456) ccw
  arc A71 (109.92, 183.8505) -> (109.92, 185.4408) centre (109.3054, 184.6456) ccw
  line L0 (146.8405, 149.59) -> (146.825, 149.59)
  line L1 (150, 149.59) -> (148.4308, 149.59)
  line L2 (146.825, 139.43) -> (146.8405, 139.43)
  line L3 (148.4308, 139.43) -> (150, 139.43)
  line L4 (146.825, 125.185) -> (146.825, 138.2213)
  line L5 (146.825, 139.4094) -> (146.825, 139.43)
  line L6 (146.825, 159.4094) -> (146.825, 159.43)
  line L7 (146.825, 150.7987) -> (146.825, 158.2213)
  line L8 (146.825, 149.59) -> (146.825, 149.6106)
  line L9 (140.08, 125.185) -> (140.1006, 125.185)
  line L10 (141.2887, 125.185) -> (146.825, 125.185)
  line L11 (148.4308, 159.43) -> (150, 159.43)
  line L12 (146.825, 159.43) -> (146.8405, 159.43)
  line L13 (140.08, 122.01) -> (140.08, 123.5792)
  line L14 (140.08, 125.1695) -> (140.08, 125.185)
  line L15 (146.8405, 169.59) -> (146.825, 169.59)
  line L16 (150, 169.59) -> (148.4308, 169.59)
  line L17 (129.92, 125.185) -> (129.92, 125.1695)
  line L18 (129.92, 123.5792) -> (129.92, 122.01)
  line L19 (146.825, 170.7987) -> (146.825, 183.835)
  line L20 (146.825, 169.59) -> (146.825, 169.6106)
  line L21 (140.08, 183.835) -> (140.1006, 183.835)
  line L22 (141.2887, 183.835) -> (146.825, 183.835)
  line L23 (120.08, 125.185) -> (120.1006, 125.185)
  line L24 (121.2887, 125.185) -> (128.7113, 125.185)
  line L25 (129.8994, 125.185) -> (129.92, 125.185)
  line L26 (140.08, 187.01) -> (140.08, 185.4408)
  line L27 (140.08, 183.8505) -> (140.08, 183.835)
  line L28 (120.08, 122.01) -> (120.08, 123.5792)
  line L29 (120.08, 125.1695) -> (120.08, 125.185)
  line L30 (129.92, 183.835) -> (129.92, 183.8505)
  line L31 (129.92, 185.4408) -> (129.92, 187.01)
  line L32 (109.92, 125.185) -> (109.92, 125.1695)
  line L33 (109.92, 123.5792) -> (109.92, 122.01)
  line L34 (120.08, 183.835) -> (120.1006, 183.835)
  line L35 (121.2887, 183.835) -> (128.7113, 183.835)
  line L36 (129.8994, 183.835) -> (129.92, 183.835)
  line L37 (100.08, 125.185) -> (100.1006, 125.185)
  line L38 (101.2887, 125.185) -> (108.7113, 125.185)
  line L39 (109.8994, 125.185) -> (109.92, 125.185)
  line L40 (120.08, 187.01) -> (120.08, 185.4408)
  line L41 (120.08, 183.8505) -> (120.08, 183.835)
  line L42 (100.08, 122.01) -> (100.08, 123.5792)
  line L43 (100.08, 125.1695) -> (100.08, 125.185)
  line L44 (109.92, 183.835) -> (109.92, 183.8505)
  line L45 (109.92, 185.4408) -> (109.92, 187.01)
  line L46 (89.92, 125.185) -> (89.92, 125.1695)
  line L47 (89.92, 123.5792) -> (89.92, 122.01)
  line L48 (100.08, 183.835) -> (100.1006, 183.835)
  line L49 (101.2887, 183.835) -> (108.7113, 183.835)
  line L50 (109.8994, 183.835) -> (109.92, 183.835)
  line L51 (80.08, 125.185) -> (80.1006, 125.185)
  line L52 (81.2887, 125.185) -> (88.7113, 125.185)
  line L53 (89.8994, 125.185) -> (89.92, 125.185)
  line L54 (100.08, 187.01) -> (100.08, 185.4408)
  line L55 (100.08, 183.8505) -> (100.08, 183.835)
  line L56 (80.08, 122.01) -> (80.08, 123.5792)
  line L57 (80.08, 125.1695) -> (80.08, 125.185)
  line L58 (89.92, 183.835) -> (89.92, 183.8505)
  line L59 (89.92, 185.4408) -> (89.92, 187.01)
  line L60 (69.92, 125.185) -> (69.92, 125.1695)
  line L61 (69.92, 123.5792) -> (69.92, 122.01)
  line L62 (80.08, 183.835) -> (80.1006, 183.835)
  line L63 (81.2887, 183.835) -> (88.7113, 183.835)
  line L64 (89.8994, 183.835) -> (89.92, 183.835)
  line L65 (60.08, 125.185) -> (60.1006, 125.185)
  line L66 (61.2887, 125.185) -> (68.7113, 125.185)
  line L67 (69.8994, 125.185) -> (69.92, 125.185)
  line L68 (80.08, 187.01) -> (80.08, 185.4408)
  line L69 (80.08, 183.8505) -> (80.08, 183.835)
  line L70 (60.08, 122.01) -> (60.08, 123.5792)
  line L71 (60.08, 125.1695) -> (60.08, 125.185)
  line L72 (69.92, 183.835) -> (69.92, 183.8505)
  line L73 (69.92, 185.4408) -> (69.92, 187.01)
  line L74 (49.92, 125.185) -> (49.92, 125.1695)
  line L75 (49.92, 123.5792) -> (49.92, 122.01)
  line L76 (60.08, 183.835) -> (60.1006, 183.835)
  line L77 (61.2887, 183.835) -> (68.7113, 183.835)
  line L78 (69.8994, 183.835) -> (69.92, 183.835)
  line L79 (40.08, 125.185) -> (40.1006, 125.185)
  line L80 (41.2887, 125.185) -> (48.7113, 125.185)
  line L81 (49.8994, 125.185) -> (49.92, 125.185)
  line L82 (60.08, 187.01) -> (60.08, 185.4408)
  line L83 (60.08, 183.8505) -> (60.08, 183.835)
  line L84 (40.08, 122.01) -> (40.08, 123.5792)
  line L85 (40.08, 125.1695) -> (40.08, 125.185)
  line L86 (49.92, 183.835) -> (49.92, 183.8505)
  line L87 (49.92, 185.4408) -> (49.92, 187.01)
  line L88 (29.92, 125.185) -> (29.92, 125.1695)
  line L89 (29.92, 123.5792) -> (29.92, 122.01)
  line L90 (40.08, 183.835) -> (40.1006, 183.835)
  line L91 (41.2887, 183.835) -> (48.7113, 183.835)
  line L92 (49.8994, 183.835) -> (49.92, 183.835)
  line L93 (20.08, 125.185) -> (20.1006, 125.185)
  line L94 (21.2887, 125.185) -> (28.7113, 125.185)
  line L95 (29.8994, 125.185) -> (29.92, 125.185)
  line L96 (40.08, 187.01) -> (40.08, 185.4408)
  line L97 (40.08, 183.8505) -> (40.08, 183.835)
  line L98 (20.08, 122.01) -> (20.08, 123.5792)
  line L99 (20.08, 125.1695) -> (20.08, 125.185)
  line L100 (29.92, 183.835) -> (29.92, 183.8505)
  line L101 (29.92, 185.4408) -> (29.92, 187.01)
  line L102 (9.92, 125.185) -> (9.92, 125.1695)
  line L103 (9.92, 123.5792) -> (9.92, 122.01)
  line L104 (3.175, 125.185) -> (8.7113, 125.185)
  line L105 (9.8994, 125.185) -> (9.92, 125.185)
  line L106 (20.08, 183.835) -> (20.1006, 183.835)
  line L107 (21.2887, 183.835) -> (28.7113, 183.835)
  line L108 (29.8994, 183.835) -> (29.92, 183.835)
  line L109 (3.175, 139.4094) -> (3.175, 139.43)
  line L110 (3.175, 125.185) -> (3.175, 138.2213)
  line L111 (20.08, 187.01) -> (20.08, 185.4408)
  line L112 (20.08, 183.8505) -> (20.08, 183.835)
  line L113 (1.5692, 139.43) -> (0, 139.43)
  line L114 (3.175, 139.43) -> (3.1595, 139.43)
  line L115 (9.92, 183.835) -> (9.92, 183.8505)
  line L116 (9.92, 185.4408) -> (9.92, 187.01)
  line L117 (3.1595, 149.59) -> (3.175, 149.59)
  line L118 (0, 149.59) -> (1.5692, 149.59)
  line L119 (3.175, 183.835) -> (8.7113, 183.835)
  line L120 (9.8994, 183.835) -> (9.92, 183.835)
  line L121 (3.175, 159.4094) -> (3.175, 159.43)
  line L122 (3.175, 150.7987) -> (3.175, 158.2213)
  line L123 (3.175, 149.59) -> (3.175, 149.6106)
  line L124 (3.175, 169.59) -> (3.175, 169.6106)
  line L125 (3.175, 170.7987) -> (3.175, 183.835)
  line L126 (1.5692, 159.43) -> (0, 159.43)
  line L127 (3.175, 159.43) -> (3.1595, 159.43)
  line L128 (0, 169.59) -> (1.5692, 169.59)
  line L129 (3.1595, 169.59) -> (3.175, 169.59)
  line L130 (0, 139.43) -> (0, 149.59)
  line L131 (0, 159.43) -> (0, 169.59)
  line L132 (9.92, 187.01) -> (20.08, 187.01)
  line L133 (29.92, 187.01) -> (40.08, 187.01)
  line L134 (49.92, 187.01) -> (60.08, 187.01)
  line L135 (69.92, 187.01) -> (80.08, 187.01)
  line L136 (89.92, 187.01) -> (100.08, 187.01)
  line L137 (109.92, 187.01) -> (120.08, 187.01)
  line L138 (129.92, 187.01) -> (140.08, 187.01)
  line L139 (150, 159.43) -> (150, 169.59)
  line L140 (150, 139.43) -> (150, 149.59)
  line L141 (129.92, 122.01) -> (140.08, 122.01)
  line L142 (109.92, 122.01) -> (120.08, 122.01)
  line L143 (89.92, 122.01) -> (100.08, 122.01)
  line L144 (69.92, 122.01) -> (80.08, 122.01)
  line L145 (49.92, 122.01) -> (60.08, 122.01)
  line L146 (29.92, 122.01) -> (40.08, 122.01)
  line L147 (9.92, 122.01) -> (20.08, 122.01)